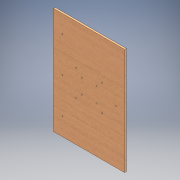
# Autodesk Inventor part: toit_robot
Saved by Autodesk Inventor 2017 (Build 210142000, 142)
## iProperties
Created: 2017-04-21
Part Number: toit_robot
Material: Generic
Document SubType Name: Modeling
Designer: franc
Density: 1 g/cm^3
Appearance: Default
Author: franc
Autodesk Inventor part; units mm, degrees
ref_plane "YZ Plane" through (0, 0, 0) normal (1, 0, 0) x (0, 1, 0)
ref_plane "XZ Plane" through (0, 0, 0) normal (0, 1, 0) x (-1, 0, 0)
ref_plane "XY Plane" through (0, 0, 0) normal (0, 0, 1) x (1, 0, 0)
sketch "Sketch1" plane through (0, 0, 0) normal (0, 1, 0) x (-1, 0, 0)
  line L0 (5.2319, 5.8808) -> (-194.7681, 5.8808)
  line L1 (-194.7681, 5.8808) -> (-194.7681, -294.1192)
  line L2 (-194.7681, -294.1192) -> (5.2319, -294.1192)
  line L3 (5.2319, -294.1192) -> (5.2319, 5.8808)
  circle A0 centre (-73.9085, -123.2596) radius 1.5
  circle A1 centre (-73.9085, -164.9789) radius 1.5
  circle A2 centre (-115.6278, -123.2596) radius 1.5
  circle A3 centre (-115.6278, -164.9789) radius 1.5
  circle A4 centre (-131.7681, -181.1192) radius 1.5
  circle A5 centre (-57.7681, -181.1192) radius 1.5
  circle A6 centre (-57.7681, -107.1192) radius 1.5
  circle A7 centre (-131.7681, -107.1192) radius 1.5
  circle A8 centre (-19.7681, -144.1192) radius 1.5
  circle A9 centre (-19.7681, -44.1192) radius 1.5
  circle A10 centre (-19.7681, -244.1192) radius 1.5
  circle A11 centre (-169.7681, -144.1192) radius 1.5
  point P0 (0, 0)
  point P1 (-94.7681, -144.1192)
  dimension "d0" = 300
  dimension "d1" = 200
  dimension "d19" = 150
  dimension "d20" = 100
  dimension "d25" = 29.5
  dimension "d26" = 29.5
  dimension "d27" = 29.5
  dimension "d28" = 29.5
  dimension "d29" = 79.1403
  dimension "d30" = 129.1404
  dimension "d31" = 79.1403
  dimension "d32" = 129.1404
  dimension "d33" = 3
  dimension "d34" = 3
  dimension "d35" = 3
  dimension "d36" = 3
  dimension "d37" = 37
  dimension "d38" = 37
  dimension "d39" = 3
  dimension "d40" = 37
  dimension "d41" = 37
  dimension "d42" = 3
  dimension "d43" = 37
  dimension "d44" = 37
  dimension "d45" = 3
  dimension "d46" = 37
  dimension "d47" = 37
  dimension "d48" = 3
  dimension "d49" = 150
  dimension "d51" = 3
  dimension "d52" = 25
  dimension "d53" = 25
  dimension "d54" = 25
  dimension "d55" = 50
  dimension "d56" = 50
  dimension "d57" = 3
  dimension "d58" = 3
  dimension "d59" = 25
  dimension "d60" = 150
  dimension "d61" = 3
  constraints: 12 centre point, 8 end point, 2 parallel, 1 horizontal, 1 perpendicular
  measures "d0" distance of L2.end L0.start
  measures "d1" distance of L0.start L0.end
  measures "d19" distance from line of L0 point (-94.768, -144.119)
  measures "d20" distance from line of L1 point (-94.768, -144.119)
  measures "d25" distance of point (-94.768, -144.119) A2.centre
  measures "d26" distance of point (-94.768, -144.119) A0.centre
  measures "d27" distance of point (-94.768, -144.119) A1.centre
  measures "d28" distance of point (-94.768, -144.119) A3.centre
  measures "d29" distance from line of L3 A1.centre
  measures "d30" distance from line of L2 A3.centre
  measures "d31" distance from line of A2.centre L1
  measures "d32" distance from line of L0 A0.centre
  measures "d33" diameter of A0
  measures "d34" diameter of A1
  measures "d35" diameter of A3
  measures "d36" diameter of A2
  measures "d37" horizontal distance of point (-94.768, -144.119) A4.centre
  measures "d38" horizontal distance of point (-94.768, -144.119) A4.centre
  measures "d39" diameter of A4
  measures "d40" horizontal distance of point (-94.768, -144.119) A5.centre
  measures "d41" horizontal distance of point (-94.768, -144.119) A5.centre
  measures "d42" diameter of A5
  measures "d43" horizontal distance of point (-94.768, -144.119) A6.centre
  measures "d44" horizontal distance of point (-94.768, -144.119) A6.centre
  measures "d45" diameter of A6
  measures "d46" horizontal distance of point (-94.768, -144.119) A7.centre
  measures "d47" horizontal distance of point (-94.768, -144.119) A7.centre
  measures "d48" diameter of A7
  measures "d49" distance from line of L0 A8.centre
  measures "d51" diameter of A8
  measures "d52" distance from line of L3 A8.centre
  measures "d53" distance from line of L3 A9.centre
  measures "d54" distance from line of L3 A10.centre
  measures "d55" distance from line of L0 A9.centre
  measures "d56" distance from line of L2 A10.centre
  measures "d57" diameter of A9
  measures "d58" diameter of A10
  measures "d59" distance from line of L1 A11.centre
  measures "d60" distance from line of L2 A11.centre
  measures "d61" diameter of A11
extrude "Extrusion1" add sketch "Sketch1" along normal blind 5
body "Solid1"
